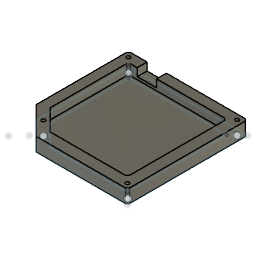
RatPad (Autodesk Fusion 360 design; units mm, degrees)
Autodesk Fusion 360 part; units mm, degrees
sketch "Sketch1" plane through (0, 0, 0) normal (0, 0, 1) x (1, 0, 0) in component "RadPad"
  line L0 (-23, 0) -> (67.25, 0)
  line L1 (69.25, -2) -> (69.25, -93.25)
  line L2 (67.25, -95.25) -> (-5, -95.25)
  line L3 (-25, -75.25) -> (-25, -2)
  line L4 (-32.5, 9.5) -> (77.75, 9.5)
  line L5 (79.75, 7.5) -> (79.75, -103.75)
  line L6 (77.75, -105.75) -> (-8, -105.75)
  line L7 (-34.5, -79.25) -> (-34.5, 7.5)
  circle A0 centre (-17.8395, -88.8395) radius 1.7
  circle A1 centre (74.75, -100.75) radius 1.7
  circle A2 centre (74.75, 4.5) radius 1.7
  circle A3 centre (-29.5, 4.5) radius 1.7
  circle A4 centre (-29.5, 4.5) radius 3
  circle A5 centre (74.75, 4.5) radius 3
  circle A6 centre (74.75, -100.75) radius 3
  circle A7 centre (-17.8395, -88.8395) radius 3
  line L8 (-25, -75.25) -> (-5, -95.25)
  line L9 (-34.5, -79.25) -> (-8, -105.75)
  line L10 (-32.5, 9.5) -> (-34.5, 7.5)
  line L11 (-25, -2) -> (-23, 0)
  line L12 (67.25, 0) -> (69.25, -2)
  line L13 (69.25, -93.25) -> (67.25, -95.25)
  line L14 (79.75, -103.75) -> (77.75, -105.75)
  line L15 (77.75, 9.5) -> (79.75, 7.5)
  point P0 (-25, 0)
  point P1 (69.25, 0)
  point P2 (69.25, -95.25)
  point P3 (-25, -95.25)
  point P4 (-34.5, 9.5)
  point P5 (79.75, 9.5)
  point P6 (79.75, -105.75)
  point P7 (-34.5, -105.75)
  point P8 (75, -100)
  dimension "d1" = 94.25
  dimension "d2" = 95.25
  dimension "d3" = 114.25
  dimension "d4" = 115.25
  dimension "d5" = 9.5
  dimension "d6" = 9.5
  dimension "d7" = 3.4
  dimension "d8" = 3.4
  dimension "d9" = 3.4
  dimension "d10" = 3.4
  dimension "d11" = 5
  dimension "d12" = 5
  dimension "d15" = 5
  dimension "d16" = 5
  dimension "d17" = 5
  dimension "d18" = 5
  dimension "d19" = 6
  dimension "d20" = 6
  dimension "d21" = 6
  dimension "d22" = 6
  dimension "d23" = 20
  dimension "d24" = 20
  dimension "d25" = 26.5
  dimension "d26" = 26.5
  dimension "d27" = 5
  dimension "d28" = 2
  dimension "d29" = 2
  dimension "d30" = 2
  dimension "d31" = 2
  dimension "d32" = 2
  dimension "d33" = 2
  dimension "d34" = 2
  dimension "d35" = 2
  dimension "d36" = 2
  dimension "d37" = 2
  dimension "d38" = 2
  dimension "d39" = 2
  constraint horizontal L0
  constraint vertical L1
  constraint horizontal L2
  constraint vertical L3
  constraint horizontal L4
  constraint vertical L5
  constraint horizontal L6
  constraint vertical L7
  constraint concentric A3 A4
  constraint concentric A2 A5
  constraint concentric A1 A6
  constraint concentric A0 A7
  constraint coincident P3 L3
  constraint coincident P3 L2
  constraint coincident P7 L7
  constraint coincident P7 L6
  constraint coincident P4 L4
  constraint coincident P4 L7
  constraint coincident P0 L3
  constraint coincident P0 L0
  constraint coincident P1 L0
  constraint coincident P1 L1
  constraint coincident P2 L1
  constraint coincident P2 L2
  constraint coincident P6 L5
  constraint coincident P6 L6
  constraint coincident P5 L4
  constraint coincident P5 L5
  measures "d1" distance of P0 P1
  measures "d2" distance of P0 P3
  measures "d3" distance of P4 P5
  measures "d4" distance of P4 P7
  measures "d5" distance of L3 L7
  measures "d6" distance of L0 L4
  measures "d7" diameter of A0
  measures "d8" diameter of A1
  measures "d9" diameter of A2
  measures "d10" diameter of A3
  measures "d11" distance of L4 A3.centre
  measures "d12" distance of L7 A3.centre
  measures "d15" distance of L6 A1.centre
  measures "d16" distance of L5 A1.centre
  measures "d17" distance of L4 A2.centre
  measures "d18" distance of L5 A2.centre
  measures "d19" diameter of A4
  measures "d20" diameter of A5
  measures "d21" diameter of A6
  measures "d22" diameter of A7
  measures "d23" distance of P3 L3.start
  measures "d24" distance of P3 L2.end
  measures "d25" distance of P7 L7.start
  measures "d26" distance of P7 L6.end
  measures "d27" distance of A0.centre L9
  measures "d28" distance of P4 L4.start
  measures "d29" distance of P4 L7.end
  measures "d30" distance of P0 L3.end
  measures "d31" distance of P0 L0.start
  measures "d32" distance of P1 L0.end
  measures "d33" distance of P1 L1.start
  measures "d34" distance of P2 L1.end
  measures "d35" distance of P2 L2.start
  measures "d36" distance of P6 L5.end
  measures "d37" distance of P6 L6.start
  measures "d38" distance of P5 L4.end
  measures "d39" distance of P5 L5.start
extrude "Extrude1" add sketch "Sketch1" along normal blind 9.9 from surface at 3.1 contours A4 | A5 | A6 | A7 makes body 1 at (75.5625, 7.3879, 9.7) makes body 2 at (77.3099, -99.1857, 9.7) makes body 3 at (-26.5037, 4.3505, 9.7) makes body 4 at (-20.3993, -90.4038, 9.7) in component "RadPad"
extrude "Extrude2" add sketch "Sketch1" along normal blind 13 contours L4 L5 L6 L7 L9 L10 L14 L15 bodies 1 2 3 4 in component "RadPad"
extrude "Extrude3" add sketch "Sketch1" along normal blind 3 contours L0 L1 L2 L3 L8 L11 L12 L13 bodies 1 in component "RadPad"
sketch "Sketch2" plane through (0, 0, 13) normal (0, 0, 1) x (-1, 0, 0) in component "RadPad"
  circle A0 centre (-74.75, -4.5) radius 1.7
  circle A1 centre (17.8395, 88.8395) radius 1.7
  line L0 (5, 95.25) -> (25, 75.25)
  line L1 (25, 75.25) -> (25, 2)
  line L2 (25, 2) -> (23, 0)
  line L3 (23, 0) -> (-67.25, 0)
  line L4 (-67.25, 0) -> (-69.25, 2)
  line L5 (-69.25, 2) -> (-69.25, 93.25)
  line L6 (-69.25, 93.25) -> (-67.25, 95.25)
  line L7 (-67.25, 95.25) -> (5, 95.25)
  line L8 (32.5, -9.5) -> (34.5, -7.5)
  line L9 (34.5, -7.5) -> (34.5, 79.25)
  line L10 (34.5, 79.25) -> (8, 105.75)
  line L11 (8, 105.75) -> (-77.75, 105.75)
  line L12 (-77.75, 105.75) -> (-79.75, 103.75)
  line L13 (-79.75, 103.75) -> (-79.75, -7.5)
  line L14 (-79.75, -7.5) -> (-77.75, -9.5)
  line L15 (-77.75, -9.5) -> (32.5, -9.5)
  circle A2 centre (-74.75, 100.75) radius 1.7
  circle A3 centre (29.5, -4.5) radius 1.7
  line L16 (16.615, -9.5) -> (-1.885, -9.5)
  line L17 (-1.885, -9.5) -> (-1.885, 0)
  line L18 (-1.885, 0) -> (16.615, 0)
  line L19 (16.615, 0) -> (16.615, -9.5)
  line L20 (34.5, 79.25) -> (34.5, -7.5)
  point P0 (25, 0)
  dimension "d47" = 18.5
  dimension "d49" = 17.885
  constraint horizontal L16
  constraint vertical L17
  constraint horizontal L18
  constraint vertical L19
  constraint coincident L15 L16.start
  measures "d47" distance of L16.start L16.end
  measures "d49" distance of L19 L20
extrude "Extrude4" cut sketch "Sketch2" against normal blind 7.5 contours L3 L15 L16 L17 L18 L19 bodies 1 in component "RadPad"
component "RadPad" placed x (1, 0, 0) y (0, 1, 0) z (0, 0, 1) at (0, 0, 0)
equation "d24 = d23"
equation "d26 = d25"
equation "d29 = d28"
equation "d31 = d30"
equation "d33 = d32"
equation "d35 = d34"
equation "d37 = d36"
equation "d39 = d38"
equation "d49 = 12.135 mm + 5.75 mm"
